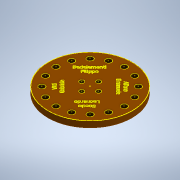
# Autodesk Inventor part: dischetto
Saved by Autodesk Inventor 2020.2 (Build 242310000, 310)
## iProperties
Created: 2020-02-12
Part Number: dischetto
Material: Legno(pioppo)
Document SubType Name: Modeling
Designer: socci
Density: 0.4 g/cm^3
Appearance: Default(1)
Mass: 18.3157 g
Surface Area: 156.78 cm^2
Volume: 45.7893 cm^3
Author: socci
Autodesk Inventor part; units mm, degrees
(part 1 of 3)
ref_plane "YZ Plane" through (0, 0, 0) normal (1, 0, 0) x (0, 1, 0)
ref_plane "XZ Plane" through (0, 0, 0) normal (0, 1, 0) x (-1, 0, 0)
ref_plane "XY Plane" through (0, 0, 0) normal (0, 0, 1) x (1, 0, 0)
sketch "Schizzo1" plane through (0, 0, 0) normal (0, 1, 0) x (-1, 0, 0)
  circle A0 centre (0, 0) radius 40
  dimension "d0" = 80
  constraints: 1 centre point, 1 coincident
  measures "d0" diameter of A0
extrude "Estrusione1" add sketch "Schizzo1" along normal blind 6
sketch "Schizzo2" plane through (0, 6, 0) normal (0, 1, 0) x (1, 0, 0)
  line L0 (0, -8) -> (0, 8)
  line L1 (0, -8) -> (16, -8) construction
  line L2 (-8, 0) -> (8, 0)
  line L3 (-8, 0) -> (8, 0) construction
  point P0 (0, 0)
  point P1 (0, 0)
  dimension "d4" = 16
  dimension "d5" = 90
  dimension "d6" = 16
  dimension "d7" = 0
  constraints: 8 end point, 3 horizontal, 2 equal length, 2 midpoint, 1 coincident, 1 vertical
  measures "d4" distance of L0.start L0.end
  measures "d5" angle of L1 L0
  measures "d6" distance of L2.start L2.end
  measures "d7" distance between parallel lines of L2 L3
hole "Foro1" at (-8, 6, 0) at (0, 6, 8) at (8, 6, 0) at (0, 6, -8) direction (0, -1, 0) diameter 4.2 end through all
sketch "Schizzo3" plane through (0, 6, 0) normal (0, 1, 0) x (1, 0, 0)
  line L0 (0, 0) -> (0, 32.5)
  point P0 (-12.4372, 30.0261)
  point P1 (-22.981, 22.981)
  point P2 (-30.0261, 12.4372)
  point P3 (-32.5, 0)
  point P4 (-30.0261, -12.4372)
  point P5 (-22.981, -22.981)
  point P6 (-12.4372, -30.0261)
  point P7 (0, -32.5)
  point P8 (12.4372, -30.0261)
  point P9 (22.981, -22.981)
  point P10 (30.0261, -12.4372)
  point P11 (32.5, 0)
  point P12 (30.0261, 12.4372)
  point P13 (22.981, 22.981)
  point P14 (12.4372, 30.0261)
  point P15 (24.3182, -23.5879)
  dimension "d15" = 32.5
  dimension "d19" = 360
  constraints: 2 end point, 1 coincident, 1 vertical, 17 other
  measures "d15" distance of L0.start L0.end
hole "Foro2" at (0, 6, -32.5) at (-30.0261, 6, 12.4372) at (-32.5, 6, 0) at (-30.0261, 6, -12.4372) at (-22.981, 6, -22.981) at (-12.4372, 6, -30.0261) at (12.4372, 6, -30.0261) at (22.981, 6, -22.981) at (30.0261, 6, -12.4372) at (32.5, 6, 0) at (30.0261, 6, 12.4372) at (22.981, 6, 22.981) at (12.4372, 6, 30.0261) at (0, 6, 32.5) at (-12.4372, 6, 30.0261) at (-22.981, 6, 22.981) direction (0, -1, 0) diameter 5.5 end through all clearance for "Vite a testa svasata piana ISO 2009/7046" size "M5" standard "ISO"
sketch "Schizzo4" plane through (0, 6, 0) normal (0, 1, 0) x (1, 0, 0)
  line L0 (-26.4914, 3.9695) -> (-4.5406, 25.9204) construction
  line L1 (-4.5406, 25.9204) -> (-2.2299, 23.6096) construction
  line L2 (-2.2299, 23.6096) -> (-24.1807, 1.6588) construction
  line L3 (-24.1807, 1.6588) -> (-26.4914, 3.9695) construction
  line L4 (9.0217, 26.78) -> (26.9135, 8.8882) construction
  line L5 (26.9135, 8.8882) -> (21.8287, 3.8034) construction
  line L6 (21.8287, 3.8034) -> (3.9369, 21.6952) construction
  line L7 (3.9369, 21.6952) -> (9.0217, 26.78) construction
  line L8 (-4.485, -26.3516) -> (-26.4359, -4.4008) construction
  line L9 (-26.4359, -4.4008) -> (-26.0745, -4.0394) construction
  line L10 (-26.0745, -4.0394) -> (-4.1237, -25.9903) construction
  line L11 (-4.1237, -25.9903) -> (-4.485, -26.3516) construction
  line L12 (23.0165, -8.2769) -> (5.176, -26.1174) construction
  line L13 (5.176, -26.1174) -> (2.8653, -23.8067) construction
  line L14 (2.8653, -23.8067) -> (20.7058, -5.9662) construction
  line L15 (20.7058, -5.9662) -> (23.0165, -8.2769) construction
  line L16 (0, 0) -> (32.9939, -32.9939) construction
  line L17 (0, 0) -> (46.6605, 0) construction
  line L18 (0, 0) -> (41.8573, 41.8573) construction
  line L19 (0, 0) -> (59.1951, 0) construction
  line L20 (0, 0) -> (-51.3067, 51.3067) construction
  line L21 (0, 0) -> (72.5586, 0) construction
  line L22 (0, 0) -> (-38.8019, -38.8019) construction
  line L23 (0, 0) -> (54.8741, 0) construction
  spline S0 degree 2 poles (-22.3396, 9.0274) (-22.1789, 8.8667) (-22.0549, 8.4981) (-22.0759, 8.3165) knots 0 0 0 1 2 2 2
  spline S1 degree 2 poles (-22.0759, 8.3165) (-22.1038, 8.0999) (-22.3012, 7.7419) (-22.5213, 7.5218) knots 0 0 0 1 2 2 2
  line L24 (-22.5213, 7.5218) -> (-23.1395, 6.9035)
  line L25 (-23.1395, 6.9035) -> (-25.2948, 9.0588)
  line L26 (-25.2948, 9.0588) -> (-24.7237, 9.6299)
  spline S2 degree 2 poles (-24.7237, 9.6299) (-24.4931, 9.8605) (-24.2329, 10.0613) (-24.0705, 10.1085) knots 0 0 0 1 2 2 2
  spline S3 degree 2 poles (-24.0705, 10.1085) (-23.8923, 10.1644) (-23.5849, 10.0701) (-23.4487, 9.9338) knots 0 0 0 1 2 2 2
  spline S4 degree 2 poles (-23.4487, 9.9338) (-23.2967, 9.7819) (-23.2164, 9.3802) (-23.2897, 9.1706) knots 0 0 0 1 2 2 2
  line L27 (-23.2897, 9.1706) -> (-23.2793, 9.1601)
  spline S5 degree 2 poles (-23.2793, 9.1601) (-23.0347, 9.2998) (-22.5457, 9.2335) (-22.3396, 9.0274) knots 0 0 0 1 2 2 2
  spline S6 degree 2 poles (-22.626, 8.7165) (-22.7483, 8.8387) (-22.9754, 8.9261) (-23.136, 8.8772) knots 0 0 0 1 2 2 2
  spline S7 degree 2 poles (-23.136, 8.8772) (-23.2391, 8.844) (-23.4207, 8.7042) (-23.5692, 8.5558) knots 0 0 0 1 2 2 2
  line L28 (-23.5692, 8.5558) -> (-23.8941, 8.2309)
  line L29 (-23.8941, 8.2309) -> (-23.0976, 7.4345)
  line L30 (-23.0976, 7.4345) -> (-22.8653, 7.6668)
  spline S8 degree 2 poles (-22.8653, 7.6668) (-22.6767, 7.8554) (-22.4951, 8.1069) (-22.4671, 8.2466) knots 0 0 0 1 2 2 2
  spline S9 degree 2 poles (-22.4671, 8.2466) (-22.4444, 8.3846) (-22.5125, 8.6029) (-22.626, 8.7165) knots 0 0 0 1 2 2 2
  spline S10 degree 2 poles (-23.7072, 9.595) (-23.784, 9.6718) (-23.9517, 9.7347) (-24.0425, 9.7103) knots 0 0 0 1 2 2 2
  spline S11 degree 2 poles (-24.0425, 9.7103) (-24.1508, 9.6788) (-24.3377, 9.5269) (-24.4896, 9.3749) knots 0 0 0 1 2 2 2
  line L31 (-24.4896, 9.3749) -> (-24.7638, 9.1007)
  line L32 (-24.7638, 9.1007) -> (-24.1333, 8.4702)
  line L33 (-24.1333, 8.4702) -> (-23.8085, 8.7951)
  spline S12 degree 2 poles (-23.8085, 8.7951) (-23.674, 8.9295) (-23.5744, 9.085) (-23.55, 9.1968) knots 0 0 0 1 2 2 2
  spline S13 degree 2 poles (-23.55, 9.1968) (-23.5255, 9.3051) (-23.6059, 9.4937) (-23.7072, 9.595) knots 0 0 0 1 2 2 2
  spline S14 degree 2 poles (-20.6839, 9.7015) (-20.6926, 9.6439) (-20.7171, 9.4448) (-20.7433, 9.3662) knots 0 0 0 1 2 2 2
  spline S15 degree 2 poles (-20.7433, 9.3662) (-20.7764, 9.2562) (-20.8708, 9.0815) (-20.993, 8.9592) knots 0 0 0 1 2 2 2
  spline S16 degree 2 poles (-20.993, 8.9592) (-21.0926, 8.8597) (-21.3476, 8.7549) (-21.4838, 8.7549) knots 0 0 0 1 2 2 2
  spline S17 degree 2 poles (-21.4838, 8.7549) (-21.6148, 8.7566) (-21.889, 8.8737) (-21.9973, 8.9819) knots 0 0 0 1 2 2 2
  spline S18 degree 2 poles (-21.9973, 8.9819) (-22.165, 9.1496) (-22.261, 9.5286) (-22.1754, 9.7504) knots 0 0 0 1 2 2 2
  spline S19 degree 2 poles (-22.1754, 9.7504) (-22.1021, 9.9495) (-21.779, 10.367) (-21.5764, 10.594) knots 0 0 0 1 2 2 2
  line L34 (-21.5764, 10.594) -> (-21.6288, 10.6464)
  spline S20 degree 2 poles (-21.6288, 10.6464) (-21.7231, 10.7407) (-21.8977, 10.8001) (-21.9833, 10.7809) knots 0 0 0 1 2 2 2
  spline S21 degree 2 poles (-21.9833, 10.7809) (-22.0689, 10.7617) (-22.2401, 10.6324) (-22.3204, 10.5521) knots 0 0 0 1 2 2 2
  spline S22 degree 2 poles (-22.3204, 10.5521) (-22.4147, 10.4578) (-22.6138, 10.1469) (-22.6872, 9.9653) knots 0 0 0 1 2 2 2
  line L35 (-22.6872, 9.9653) -> (-22.7029, 9.9495)
  line L36 (-22.7029, 9.9495) -> (-22.9806, 10.2272)
  spline S23 degree 2 poles (-22.9806, 10.2272) (-22.9265, 10.3233) (-22.6977, 10.6569) (-22.5597, 10.7949) knots 0 0 0 1 2 2 2
  spline S24 degree 2 poles (-22.5597, 10.7949) (-22.392, 10.9626) (-22.1108, 11.139) (-21.9519, 11.1617) knots 0 0 0 1 2 2 2
  spline S25 degree 2 poles (-21.9519, 11.1617) (-21.7964, 11.1844) (-21.4978, 11.0604) (-21.3458, 10.9084) knots 0 0 0 1 2 2 2
  line L37 (-21.3458, 10.9084) -> (-20.2402, 9.8028)
  line L38 (-20.2402, 9.8028) -> (-20.5127, 9.5304)
  line L39 (-20.5127, 9.5304) -> (-20.6839, 9.7015)
  line L40 (-20.9109, 9.9286) -> (-21.3598, 10.3775)
  spline S26 degree 2 poles (-21.3598, 10.3775) (-21.4489, 10.2709) (-21.7143, 9.946) (-21.779, 9.8255) knots 0 0 0 1 2 2 2
  spline S27 degree 2 poles (-21.779, 9.8255) (-21.8541, 9.6841) (-21.8576, 9.4046) (-21.7353, 9.2824) knots 0 0 0 1 2 2 2
  spline S28 degree 2 poles (-21.7353, 9.2824) (-21.5956, 9.1426) (-21.2969, 9.1583) (-21.1467, 9.3086) knots 0 0 0 1 2 2 2
  spline S29 degree 2 poles (-21.1467, 9.3086) (-21.0192, 9.4361) (-20.9197, 9.7557) (-20.9109, 9.9286) knots 0 0 0 1 2 2 2
  line L41 (-18.6142, 11.4289) -> (-18.8867, 11.1564)
  line L42 (-18.8867, 11.1564) -> (-19.0508, 11.3206)
  spline S30 degree 2 poles (-19.0508, 11.3206) (-19.0613, 11.2053) (-19.084, 11.0429) (-19.1172, 10.9503) knots 0 0 0 1 2 2 2
  spline S31 degree 2 poles (-19.1172, 10.9503) (-19.1469, 10.8647) (-19.2412, 10.711) (-19.3233, 10.629) knots 0 0 0 1 2 2 2
  spline S32 degree 2 poles (-19.3233, 10.629) (-19.456, 10.4962) (-19.7896, 10.3827) (-19.9748, 10.4106) knots 0 0 0 1 2 2 2
  spline S33 degree 2 poles (-19.9748, 10.4106) (-20.1599, 10.4386) (-20.5616, 10.6656) (-20.766, 10.87) knots 0 0 0 1 2 2 2
  spline S34 degree 2 poles (-20.766, 10.87) (-20.979, 11.0831) (-21.1799, 11.504) (-21.2009, 11.7171) knots 0 0 0 1 2 2 2
  spline S35 degree 2 poles (-21.2009, 11.7171) (-21.2166, 11.9109) (-21.0873, 12.2812) (-20.9493, 12.4192) knots 0 0 0 1 2 2 2
  spline S36 degree 2 poles (-20.9493, 12.4192) (-20.8288, 12.5397) (-20.5948, 12.6655) (-20.4394, 12.7091) knots 0 0 0 1 2 2 2
  line L43 (-20.4394, 12.7091) -> (-21.138, 13.4077)
  line L44 (-21.138, 13.4077) -> (-20.8655, 13.6802)
  line L45 (-20.8655, 13.6802) -> (-18.6142, 11.4289)
  line L46 (-19.2796, 11.5494) -> (-20.214, 12.4838)
  spline S37 degree 2 poles (-20.214, 12.4838) (-20.3642, 12.4314) (-20.5616, 12.3074) (-20.6542, 12.2148) knots 0 0 0 1 2 2 2
  spline S38 degree 2 poles (-20.6542, 12.2148) (-20.8638, 12.0052) (-20.7869, 11.4533) (-20.49, 11.1564) knots 0 0 0 1 2 2 2
  spline S39 degree 2 poles (-20.49, 11.1564) (-20.2036, 10.87) (-19.7198, 10.7495) (-19.5189, 10.9503) knots 0 0 0 1 2 2 2
  spline S40 degree 2 poles (-19.5189, 10.9503) (-19.4124, 11.0569) (-19.2936, 11.3712) (-19.2796, 11.5494) knots 0 0 0 1 2 2 2
  spline S41 degree 2 poles (-17.4894, 12.896) (-17.4981, 12.8384) (-17.5226, 12.6393) (-17.5488, 12.5607) knots 0 0 0 1 2 2 2
  spline S42 degree 2 poles (-17.5488, 12.5607) (-17.582, 12.4506) (-17.6763, 12.276) (-17.7985, 12.1537) knots 0 0 0 1 2 2 2
  spline S43 degree 2 poles (-17.7985, 12.1537) (-17.8981, 12.0542) (-18.1531, 11.9494) (-18.2893, 11.9494) knots 0 0 0 1 2 2 2
  spline S44 degree 2 poles (-18.2893, 11.9494) (-18.4203, 11.9511) (-18.6945, 12.0681) (-18.8028, 12.1764) knots 0 0 0 1 2 2 2
  spline S45 degree 2 poles (-18.8028, 12.1764) (-18.9705, 12.3441) (-19.0665, 12.7231) (-18.981, 12.9449) knots 0 0 0 1 2 2 2
  spline S46 degree 2 poles (-18.981, 12.9449) (-18.9076, 13.144) (-18.5845, 13.5614) (-18.3819, 13.7885) knots 0 0 0 1 2 2 2
  line L47 (-18.3819, 13.7885) -> (-18.4343, 13.8409)
  spline S47 degree 2 poles (-18.4343, 13.8409) (-18.5286, 13.9352) (-18.7033, 13.9946) (-18.7888, 13.9754) knots 0 0 0 1 2 2 2
  spline S48 degree 2 poles (-18.7888, 13.9754) (-18.8744, 13.9562) (-19.0456, 13.8269) (-19.1259, 13.7466) knots 0 0 0 1 2 2 2
  spline S49 degree 2 poles (-19.1259, 13.7466) (-19.2202, 13.6523) (-19.4194, 13.3414) (-19.4927, 13.1597) knots 0 0 0 1 2 2 2
  line L48 (-19.4927, 13.1597) -> (-19.5084, 13.144)
  line L49 (-19.5084, 13.144) -> (-19.7861, 13.4217)
  spline S50 degree 2 poles (-19.7861, 13.4217) (-19.732, 13.5178) (-19.5032, 13.8514) (-19.3652, 13.9893) knots 0 0 0 1 2 2 2
  spline S51 degree 2 poles (-19.3652, 13.9893) (-19.1975, 14.157) (-18.9163, 14.3334) (-18.7574, 14.3561) knots 0 0 0 1 2 2 2
  spline S52 degree 2 poles (-18.7574, 14.3561) (-18.602, 14.3788) (-18.3033, 14.2548) (-18.1513, 14.1029) knots 0 0 0 1 2 2 2
  line L50 (-18.1513, 14.1029) -> (-17.0458, 12.9973)
  line L51 (-17.0458, 12.9973) -> (-17.3182, 12.7248)
  line L52 (-17.3182, 12.7248) -> (-17.4894, 12.896)
  line L53 (-17.7165, 13.1231) -> (-18.1653, 13.5719)
  spline S53 degree 2 poles (-18.1653, 13.5719) (-18.2544, 13.4654) (-18.5199, 13.1405) (-18.5845, 13.02) knots 0 0 0 1 2 2 2
  spline S54 degree 2 poles (-18.5845, 13.02) (-18.6596, 12.8785) (-18.6631, 12.5991) (-18.5408, 12.4768) knots 0 0 0 1 2 2 2
  spline S55 degree 2 poles (-18.5408, 12.4768) (-18.4011, 12.3371) (-18.1024, 12.3528) (-17.9522, 12.503) knots 0 0 0 1 2 2 2
  spline S56 degree 2 poles (-17.9522, 12.503) (-17.8247, 12.6305) (-17.7252, 12.9501) (-17.7165, 13.1231) knots 0 0 0 1 2 2 2
  line L54 (-16.3856, 13.6575) -> (-16.658, 13.385)
  line L55 (-16.658, 13.385) -> (-18.9094, 15.6364)
  line L56 (-18.9094, 15.6364) -> (-18.6369, 15.9088)
  line L57 (-18.6369, 15.9088) -> (-16.3856, 13.6575)
  spline S57 degree 2 poles (-15.2555, 15.1299) (-15.2643, 15.0722) (-15.2887, 14.8731) (-15.3149, 14.7945) knots 0 0 0 1 2 2 2
  spline S58 degree 2 poles (-15.3149, 14.7945) (-15.3481, 14.6845) (-15.4424, 14.5098) (-15.5647, 14.3876) knots 0 0 0 1 2 2 2
  spline S59 degree 2 poles (-15.5647, 14.3876) (-15.6642, 14.288) (-15.9192, 14.1832) (-16.0555, 14.1832) knots 0 0 0 1 2 2 2
  spline S60 degree 2 poles (-16.0555, 14.1832) (-16.1865, 14.185) (-16.4607, 14.302) (-16.569, 14.4103) knots 0 0 0 1 2 2 2
  spline S61 degree 2 poles (-16.569, 14.4103) (-16.7366, 14.5779) (-16.8327, 14.9569) (-16.7471, 15.1788) knots 0 0 0 1 2 2 2
  spline S62 degree 2 poles (-16.7471, 15.1788) (-16.6738, 15.3779) (-16.3506, 15.7953) (-16.148, 16.0223) knots 0 0 0 1 2 2 2
  line L58 (-16.148, 16.0223) -> (-16.2004, 16.0747)
  spline S63 degree 2 poles (-16.2004, 16.0747) (-16.2948, 16.1691) (-16.4694, 16.2284) (-16.555, 16.2092) knots 0 0 0 1 2 2 2
  spline S64 degree 2 poles (-16.555, 16.2092) (-16.6406, 16.19) (-16.8117, 16.0608) (-16.8921, 15.9804) knots 0 0 0 1 2 2 2
  spline S65 degree 2 poles (-16.8921, 15.9804) (-16.9864, 15.8861) (-17.1855, 15.5752) (-17.2589, 15.3936) knots 0 0 0 1 2 2 2
  line L59 (-17.2589, 15.3936) -> (-17.2746, 15.3779)
  line L60 (-17.2746, 15.3779) -> (-17.5523, 15.6556)
  spline S66 degree 2 poles (-17.5523, 15.6556) (-17.4981, 15.7516) (-17.2693, 16.0852) (-17.1314, 16.2232) knots 0 0 0 1 2 2 2
  spline S67 degree 2 poles (-17.1314, 16.2232) (-16.9637, 16.3909) (-16.6825, 16.5673) (-16.5236, 16.59) knots 0 0 0 1 2 2 2
  spline S68 degree 2 poles (-16.5236, 16.59) (-16.3681, 16.6127) (-16.0694, 16.4887) (-15.9175, 16.3367) knots 0 0 0 1 2 2 2
  line L61 (-15.9175, 16.3367) -> (-14.8119, 15.2312)
  line L62 (-14.8119, 15.2312) -> (-15.0844, 14.9587)
  line L63 (-15.0844, 14.9587) -> (-15.2555, 15.1299)
  line L64 (-15.4826, 15.3569) -> (-15.9315, 15.8058)
  spline S69 degree 2 poles (-15.9315, 15.8058) (-16.0205, 15.6992) (-16.286, 15.3744) (-16.3506, 15.2539) knots 0 0 0 1 2 2 2
  spline S70 degree 2 poles (-16.3506, 15.2539) (-16.4257, 15.1124) (-16.4292, 14.8329) (-16.307, 14.7107) knots 0 0 0 1 2 2 2
  spline S71 degree 2 poles (-16.307, 14.7107) (-16.1673, 14.571) (-15.8686, 14.5867) (-15.7184, 14.7369) knots 0 0 0 1 2 2 2
  spline S72 degree 2 poles (-15.7184, 14.7369) (-15.5909, 14.8644) (-15.4913, 15.184) (-15.4826, 15.3569) knots 0 0 0 1 2 2 2
  line L65 (-12.5955, 17.4475) -> (-13.5317, 18.3837)
  spline S73 degree 2 poles (-13.5317, 18.3837) (-13.6435, 18.4955) (-13.8513, 18.6684) (-13.9316, 18.6928) knots 0 0 0 1 2 2 2
  spline S74 degree 2 poles (-13.9316, 18.6928) (-14.0172, 18.7225) (-14.1797, 18.6719) (-14.2722, 18.5793) knots 0 0 0 1 2 2 2
  spline S75 degree 2 poles (-14.2722, 18.5793) (-14.3561, 18.4955) (-14.4451, 18.2003) (-14.4486, 18.0012) knots 0 0 0 1 2 2 2
  spline S76 degree 2 poles (-14.4486, 18.0012) (-14.4224, 17.9785) (-14.3508, 17.9139) (-14.3054, 17.8685) knots 0 0 0 1 2 2 2
  line L66 (-14.3054, 17.8685) -> (-13.24, 16.8031)
  line L67 (-13.24, 16.8031) -> (-13.5125, 16.5306)
  line L68 (-13.5125, 16.5306) -> (-14.4486, 17.4668)
  spline S77 degree 2 poles (-14.4486, 17.4668) (-14.5604, 17.5785) (-14.7683, 17.7514) (-14.8486, 17.7759) knots 0 0 0 1 2 2 2
  spline S78 degree 2 poles (-14.8486, 17.7759) (-14.9342, 17.8056) (-15.0966, 17.7549) (-15.1892, 17.6624) knots 0 0 0 1 2 2 2
  spline S79 degree 2 poles (-15.1892, 17.6624) (-15.2765, 17.575) (-15.3603, 17.2711) (-15.3656, 17.0947) knots 0 0 0 1 2 2 2
  line L69 (-15.3656, 17.0947) -> (-14.157, 15.8861)
  line L70 (-14.157, 15.8861) -> (-14.4294, 15.6137)
  line L71 (-14.4294, 15.6137) -> (-16.0467, 17.231)
  line L72 (-16.0467, 17.231) -> (-15.7743, 17.5034)
  line L73 (-15.7743, 17.5034) -> (-15.5961, 17.3253)
  spline S80 degree 2 poles (-15.5961, 17.3253) (-15.5961, 17.5384) (-15.5036, 17.865) (-15.3778, 17.9907) knots 0 0 0 1 2 2 2
  spline S81 degree 2 poles (-15.3778, 17.9907) (-15.2346, 18.1339) (-14.8818, 18.2248) (-14.6757, 18.1339) knots 0 0 0 1 2 2 2
  spline S82 degree 2 poles (-14.6757, 18.1339) (-14.6897, 18.3959) (-14.5971, 18.7714) (-14.4609, 18.9077) knots 0 0 0 1 2 2 2
  spline S83 degree 2 poles (-14.4609, 18.9077) (-14.3561, 19.0125) (-14.1203, 19.119) (-13.984, 19.1085) knots 0 0 0 1 2 2 2
  spline S84 degree 2 poles (-13.984, 19.1085) (-13.8461, 19.0998) (-13.5544, 18.9513) (-13.3885, 18.7854) knots 0 0 0 1 2 2 2
  line L74 (-13.3885, 18.7854) -> (-12.3231, 17.72)
  line L75 (-12.3231, 17.72) -> (-12.5955, 17.4475)
  spline S85 degree 2 poles (-11.2018, 18.768) (-11.5895, 18.3802) (-12.4506, 18.3889) (-12.8523, 18.7907) knots 0 0 0 1 2 2 2
  spline S86 degree 2 poles (-12.8523, 18.7907) (-13.247, 19.1854) (-13.3011, 20.0674) (-12.9675, 20.401) knots 0 0 0 1 2 2 2
  spline S87 degree 2 poles (-12.9675, 20.401) (-12.8173, 20.5512) (-12.4977, 20.6962) (-12.3196, 20.6892) knots 0 0 0 1 2 2 2
  spline S88 degree 2 poles (-12.3196, 20.6892) (-12.1397, 20.6839) (-11.7799, 20.5093) (-11.586, 20.3154) knots 0 0 0 1 2 2 2
  line L76 (-11.586, 20.3154) -> (-11.4376, 20.1669)
  line L77 (-11.4376, 20.1669) -> (-12.5571, 19.0474)
  spline S89 degree 2 poles (-12.5571, 19.0474) (-12.2759, 18.7662) (-11.6943, 18.7505) (-11.4428, 19.002) knots 0 0 0 1 2 2 2
  spline S90 degree 2 poles (-11.4428, 19.002) (-11.3537, 19.0911) (-11.221, 19.3041) (-11.1826, 19.4054) knots 0 0 0 1 2 2 2
  spline S91 degree 2 poles (-11.1826, 19.4054) (-11.1441, 19.5137) (-11.104, 19.6762) (-11.0987, 19.7373) knots 0 0 0 1 2 2 2
  line L78 (-11.0987, 19.7373) -> (-11.083, 19.753)
  line L79 (-11.083, 19.753) -> (-10.7861, 19.4561)
  spline S92 degree 2 poles (-10.7861, 19.4561) (-10.814, 19.3897) (-10.9014, 19.1906) (-10.9415, 19.119) knots 0 0 0 1 2 2 2
  spline S93 degree 2 poles (-10.9415, 19.119) (-10.9974, 19.0177) (-11.104, 18.8658) (-11.2018, 18.768) knots 0 0 0 1 2 2 2
  spline S94 degree 2 poles (-11.9109, 20.1093) (-12.0244, 20.2159) (-12.2305, 20.3311) (-12.3283, 20.3416) knots 0 0 0 1 2 2 2
  spline S95 degree 2 poles (-12.3283, 20.3416) (-12.4366, 20.3556) (-12.6497, 20.2717) (-12.7597, 20.1617) knots 0 0 0 1 2 2 2
  spline S96 degree 2 poles (-12.7597, 20.1617) (-12.868, 20.0534) (-12.9553, 19.8368) (-12.9553, 19.7111) knots 0 0 0 1 2 2 2
  spline S97 degree 2 poles (-12.9553, 19.7111) (-12.9518, 19.5853) (-12.8593, 19.367) (-12.7649, 19.2552) knots 0 0 0 1 2 2 2
  line L80 (-12.7649, 19.2552) -> (-11.9109, 20.1093)
  line L81 (-9.1111, 20.9319) -> (-9.3836, 20.6595)
  line L82 (-9.3836, 20.6595) -> (-10.3058, 21.5817)
  spline S98 degree 2 poles (-10.3058, 21.5817) (-10.4176, 21.6934) (-10.6306, 21.8646) (-10.7197, 21.8908) knots 0 0 0 1 2 2 2
  spline S99 degree 2 poles (-10.7197, 21.8908) (-10.814, 21.9188) (-10.9922, 21.8594) (-11.0935, 21.7581) knots 0 0 0 1 2 2 2
  spline S100 degree 2 poles (-11.0935, 21.7581) (-11.1948, 21.6568) (-11.3013, 21.3337) (-11.317, 21.1433) knots 0 0 0 1 2 2 2
  line L83 (-11.317, 21.1433) -> (-10.1084, 19.9347)
  line L84 (-10.1084, 19.9347) -> (-10.3809, 19.6622)
  line L85 (-10.3809, 19.6622) -> (-11.9982, 21.2795)
  line L86 (-11.9982, 21.2795) -> (-11.7257, 21.552)
  line L87 (-11.7257, 21.552) -> (-11.5458, 21.3721)
  spline S101 degree 2 poles (-11.5458, 21.3721) (-11.5336, 21.6044) (-11.4131, 21.9554) (-11.2804, 22.0882) knots 0 0 0 1 2 2 2
  spline S102 degree 2 poles (-11.2804, 22.0882) (-11.0428, 22.3257) (-10.4595, 22.2803) (-10.1608, 21.9816) knots 0 0 0 1 2 2 2
  line L88 (-10.1608, 21.9816) -> (-9.1111, 20.9319)
  spline S103 degree 2 poles (-8.2082, 21.772) (-8.43, 21.5502) (-8.933, 21.5537) (-9.2072, 21.8279) knots 0 0 0 1 2 2 2
  line L89 (-9.2072, 21.8279) -> (-10.1032, 22.7239)
  line L90 (-10.1032, 22.7239) -> (-10.2866, 22.5405)
  line L91 (-10.2866, 22.5405) -> (-10.5119, 22.7658)
  line L92 (-10.5119, 22.7658) -> (-10.3285, 22.9492)
  line L93 (-10.3285, 22.9492) -> (-10.7931, 23.4138)
  line L94 (-10.7931, 23.4138) -> (-10.5206, 23.6863)
  line L95 (-10.5206, 23.6863) -> (-10.056, 23.2217)
  line L96 (-10.056, 23.2217) -> (-9.5548, 23.723)
  line L97 (-9.5548, 23.723) -> (-9.3294, 23.4976)
  line L98 (-9.3294, 23.4976) -> (-9.8307, 22.9964)
  line L99 (-9.8307, 22.9964) -> (-9.0605, 22.2261)
  spline S104 degree 2 poles (-9.0605, 22.2261) (-8.9382, 22.1039) (-8.795, 21.9781) (-8.7077, 21.9502) knots 0 0 0 1 2 2 2
  spline S105 degree 2 poles (-8.7077, 21.9502) (-8.6326, 21.924) (-8.4719, 21.9834) (-8.3776, 22.0777) knots 0 0 0 1 2 2 2
  spline S106 degree 2 poles (-8.3776, 22.0777) (-8.3112, 22.1441) (-8.2274, 22.3082) (-8.2116, 22.3484) knots 0 0 0 1 2 2 2
  line L100 (-8.2116, 22.3484) -> (-8.1959, 22.3641)
  line L101 (-8.1959, 22.3641) -> (-7.9514, 22.1196)
  spline S107 degree 2 poles (-7.9514, 22.1196) (-8.0073, 22.0218) (-8.14, 21.8402) (-8.2082, 21.772) knots 0 0 0 1 2 2 2
  line L102 (-7.4589, 22.5842) -> (-7.7313, 22.3117)
  line L103 (-7.7313, 22.3117) -> (-9.3487, 23.9291)
  line L104 (-9.3487, 23.9291) -> (-9.0762, 24.2015)
  line L105 (-9.0762, 24.2015) -> (-7.4589, 22.5842)
  line L106 (-9.326, 24.4897) -> (-9.6351, 24.1806)
  line L107 (-9.6351, 24.1806) -> (-9.918, 24.4635)
  line L108 (-9.918, 24.4635) -> (-9.6089, 24.7726)
  line L109 (-9.6089, 24.7726) -> (-9.326, 24.4897)
  line L110 (-16.3834, 10.363) -> (-17.3859, 9.3605)
  line L111 (-17.3859, 9.3605) -> (-16.7781, 8.7527)
  line L112 (-16.7781, 8.7527) -> (-15.8175, 9.7133)
  line L113 (-15.8175, 9.7133) -> (-15.5625, 9.4583)
  line L114 (-15.5625, 9.4583) -> (-16.5231, 8.4977)
  line L115 (-16.5231, 8.4977) -> (-15.4857, 7.4603)
  line L116 (-15.4857, 7.4603) -> (-15.7721, 7.1738)
  line L117 (-15.7721, 7.1738) -> (-17.9274, 9.3291)
  line L118 (-17.9274, 9.3291) -> (-16.6384, 10.618)
  line L119 (-16.6384, 10.618) -> (-16.3834, 10.363)
  line L120 (-13.9696, 8.9763) -> (-14.2421, 8.7038)
  line L121 (-14.2421, 8.7038) -> (-15.8594, 10.3211)
  line L122 (-15.8594, 10.3211) -> (-15.587, 10.5936)
  line L123 (-15.587, 10.5936) -> (-13.9696, 8.9763)
  line L124 (-15.8367, 10.8818) -> (-16.1459, 10.5726)
  line L125 (-16.1459, 10.5726) -> (-16.4288, 10.8556)
  line L126 (-16.4288, 10.8556) -> (-16.1197, 11.1647)
  line L127 (-16.1197, 11.1647) -> (-15.8367, 10.8818)
  line L128 (-13.292, 9.6539) -> (-13.5644, 9.3815)
  line L129 (-13.5644, 9.3815) -> (-15.8158, 11.6328)
  line L130 (-15.8158, 11.6328) -> (-15.5433, 11.9053)
  line L131 (-15.5433, 11.9053) -> (-13.292, 9.6539)
  line L132 (-12.6143, 10.3316) -> (-12.8868, 10.0591)
  line L133 (-12.8868, 10.0591) -> (-14.5041, 11.6765)
  line L134 (-14.5041, 11.6765) -> (-14.2316, 11.9489)
  line L135 (-14.2316, 11.9489) -> (-12.6143, 10.3316)
  line L136 (-14.4814, 12.2371) -> (-14.7905, 11.928)
  line L137 (-14.7905, 11.928) -> (-15.0735, 12.2109)
  line L138 (-15.0735, 12.2109) -> (-14.7643, 12.5201)
  line L139 (-14.7643, 12.5201) -> (-14.4814, 12.2371)
  spline S108 degree 2 poles (-11.7113, 12.9392) (-11.3061, 12.534) (-11.2136, 11.6695) (-11.5087, 11.3743) knots 0 0 0 1 2 2 2
  spline S109 degree 2 poles (-11.5087, 11.3743) (-11.6292, 11.2538) (-11.8703, 11.1245) (-12.024, 11.0861) knots 0 0 0 1 2 2 2
  line L140 (-12.024, 11.0861) -> (-11.3463, 10.4085)
  line L141 (-11.3463, 10.4085) -> (-11.6188, 10.136)
  line L142 (-11.6188, 10.136) -> (-13.8317, 12.3489)
  line L143 (-13.8317, 12.3489) -> (-13.5592, 12.6214)
  line L144 (-13.5592, 12.6214) -> (-13.3898, 12.4519)
  spline S110 degree 2 poles (-13.3898, 12.4519) (-13.381, 12.6458) (-13.2553, 13.0161) (-13.1103, 13.161) knots 0 0 0 1 2 2 2
  spline S111 degree 2 poles (-13.1103, 13.161) (-12.8326, 13.4387) (-12.0816, 13.3095) (-11.7113, 12.9392) knots 0 0 0 1 2 2 2
  spline S112 degree 2 poles (-11.9611, 12.6266) (-12.2388, 12.9043) (-12.7208, 13.0335) (-12.9182, 12.8362) knots 0 0 0 1 2 2 2
  spline S113 degree 2 poles (-12.9182, 12.8362) (-13.0335, 12.7209) (-13.147, 12.4013) (-13.1627, 12.2249) knots 0 0 0 1 2 2 2
  line L145 (-13.1627, 12.2249) -> (-12.244, 11.3062)
  spline S114 degree 2 poles (-12.244, 11.3062) (-12.0868, 11.3621) (-11.8965, 11.4756) (-11.7987, 11.5734) knots 0 0 0 1 2 2 2
  spline S115 degree 2 poles (-11.7987, 11.5734) (-11.5873, 11.7847) (-11.6642, 12.3297) (-11.9611, 12.6266) knots 0 0 0 1 2 2 2
  spline S116 degree 2 poles (-10.0731, 14.5775) (-9.6678, 14.1723) (-9.5753, 13.3078) (-9.8704, 13.0126) knots 0 0 0 1 2 2 2
  spline S117 degree 2 poles (-9.8704, 13.0126) (-9.991, 12.8921) (-10.232, 12.7628) (-10.3857, 12.7244) knots 0 0 0 1 2 2 2
  line L146 (-10.3857, 12.7244) -> (-9.708, 12.0467)
  line L147 (-9.708, 12.0467) -> (-9.9805, 11.7743)
  line L148 (-9.9805, 11.7743) -> (-12.1934, 13.9872)
  line L149 (-12.1934, 13.9872) -> (-11.9209, 14.2596)
  line L150 (-11.9209, 14.2596) -> (-11.7515, 14.0902)
  spline S118 degree 2 poles (-11.7515, 14.0902) (-11.7428, 14.2841) (-11.617, 14.6544) (-11.4721, 14.7993) knots 0 0 0 1 2 2 2
  spline S119 degree 2 poles (-11.4721, 14.7993) (-11.1943, 15.077) (-10.4433, 14.9478) (-10.0731, 14.5775) knots 0 0 0 1 2 2 2
  spline S120 degree 2 poles (-10.3228, 14.2649) (-10.6005, 14.5426) (-11.0826, 14.6718) (-11.2799, 14.4745) knots 0 0 0 1 2 2 2
  spline S121 degree 2 poles (-11.2799, 14.4745) (-11.3952, 14.3592) (-11.5087, 14.0396) (-11.5244, 13.8632) knots 0 0 0 1 2 2 2
  line L151 (-11.5244, 13.8632) -> (-10.6058, 12.9445)
  spline S122 degree 2 poles (-10.6058, 12.9445) (-10.4486, 13.0004) (-10.2582, 13.1139) (-10.1604, 13.2117) knots 0 0 0 1 2 2 2
  spline S123 degree 2 poles (-10.1604, 13.2117) (-9.949, 13.423) (-10.0259, 13.968) (-10.3228, 14.2649) knots 0 0 0 1 2 2 2
  spline S124 degree 2 poles (-8.4173, 16.1459) (-8.0086, 15.7372) (-7.9562, 14.8989) (-8.2846, 14.5705) knots 0 0 0 1 2 2 2
  spline S125 degree 2 poles (-8.2846, 14.5705) (-8.6217, 14.2334) (-9.467, 14.3068) (-9.8617, 14.7015) knots 0 0 0 1 2 2 2
  spline S126 degree 2 poles (-9.8617, 14.7015) (-10.2669, 15.1067) (-10.3176, 15.9538) (-9.9927, 16.2787) knots 0 0 0 1 2 2 2
  spline S127 degree 2 poles (-9.9927, 16.2787) (-9.6644, 16.607) (-8.8243, 16.5529) (-8.4173, 16.1459) knots 0 0 0 1 2 2 2
  spline S128 degree 2 poles (-8.6985, 15.8647) (-9.0129, 16.1791) (-9.5473, 16.256) (-9.7587, 16.0446) knots 0 0 0 1 2 2 2
  spline S129 degree 2 poles (-9.7587, 16.0446) (-9.97, 15.8333) (-9.8949, 15.2971) (-9.5805, 14.9827) knots 0 0 0 1 2 2 2
  spline S130 degree 2 poles (-9.5805, 14.9827) (-9.2749, 14.6771) (-8.7299, 14.5932) (-8.5186, 14.8046) knots 0 0 0 1 2 2 2
  spline S131 degree 2 poles (-8.5186, 14.8046) (-8.309, 15.0141) (-8.3876, 15.5538) (-8.6985, 15.8647) knots 0 0 0 1 2 2 2
  line L152 (11.9676, 20.078) -> (14.8495, 21.5066)
  line L153 (14.8495, 21.5066) -> (15.2023, 21.1538)
  line L154 (15.2023, 21.1538) -> (13.7736, 18.272)
  line L155 (13.7736, 18.272) -> (13.4714, 18.5742)
  line L156 (13.4714, 18.5742) -> (13.8784, 19.3723)
  line L157 (13.8784, 19.3723) -> (13.0558, 20.195)
  line L158 (13.0558, 20.195) -> (12.2576, 19.788)
  line L159 (12.2576, 19.788) -> (11.9676, 20.078)
  line L160 (14.0443, 19.6955) -> (14.7255, 21.0438)
  line L161 (14.7255, 21.0438) -> (13.3789, 20.3609)
  line L162 (13.3789, 20.3609) -> (14.0443, 19.6955)
  line L163 (14.2347, 17.8109) -> (13.9622, 18.0834)
  line L164 (13.9622, 18.0834) -> (16.2135, 20.3347)
  line L165 (16.2135, 20.3347) -> (16.486, 20.0622)
  line L166 (16.486, 20.0622) -> (14.2347, 17.8109)
  line L167 (17.4746, 18.5497) -> (17.4606, 18.5637)
  spline S132 degree 2 poles (17.4606, 18.5637) (17.4379, 18.6143) (17.3261, 18.775) (17.272, 18.8292) knots 0 0 0 1 2 2 2
  spline S133 degree 2 poles (17.272, 18.8292) (17.1008, 19.0003) (16.8004, 18.9933) (16.5978, 18.7907) knots 0 0 0 1 2 2 2
  line L168 (16.5978, 18.7907) -> (16.5436, 18.7366)
  line L169 (16.5436, 18.7366) -> (16.9943, 18.286)
  line L170 (16.9943, 18.286) -> (16.7689, 18.0607)
  line L171 (16.7689, 18.0607) -> (16.3271, 18.5025)
  line L172 (16.3271, 18.5025) -> (14.9351, 17.1105)
  line L173 (14.9351, 17.1105) -> (14.6626, 17.383)
  line L174 (14.6626, 17.383) -> (16.0546, 18.775)
  line L175 (16.0546, 18.775) -> (15.8712, 18.9584)
  line L176 (15.8712, 18.9584) -> (16.0965, 19.1837)
  line L177 (16.0965, 19.1837) -> (16.2799, 19.0003)
  line L178 (16.2799, 19.0003) -> (16.3341, 19.0545)
  spline S134 degree 2 poles (16.3341, 19.0545) (16.624, 19.3444) (17.2091, 19.3671) (17.4711, 19.1051) knots 0 0 0 1 2 2 2
  spline S135 degree 2 poles (17.4711, 19.1051) (17.5462, 19.03) (17.6754, 18.8693) (17.7243, 18.7995) knots 0 0 0 1 2 2 2
  line L179 (17.7243, 18.7995) -> (17.4746, 18.5497)
  spline S136 degree 2 poles (16.6502, 15.7377) (16.5925, 15.7465) (16.3934, 15.7709) (16.3148, 15.7971) knots 0 0 0 1 2 2 2
  spline S137 degree 2 poles (16.3148, 15.7971) (16.2048, 15.8303) (16.0302, 15.9246) (15.9079, 16.0469) knots 0 0 0 1 2 2 2
  spline S138 degree 2 poles (15.9079, 16.0469) (15.8083, 16.1464) (15.7035, 16.4014) (15.7035, 16.5377) knots 0 0 0 1 2 2 2
  spline S139 degree 2 poles (15.7035, 16.5377) (15.7053, 16.6687) (15.8223, 16.9429) (15.9306, 17.0512) knots 0 0 0 1 2 2 2
  spline S140 degree 2 poles (15.9306, 17.0512) (16.0983, 17.2188) (16.4773, 17.3149) (16.6991, 17.2293) knots 0 0 0 1 2 2 2
  spline S141 degree 2 poles (16.6991, 17.2293) (16.8982, 17.1559) (17.3156, 16.8328) (17.5427, 16.6302) knots 0 0 0 1 2 2 2
  line L180 (17.5427, 16.6302) -> (17.5951, 16.6826)
  spline S142 degree 2 poles (17.5951, 16.6826) (17.6894, 16.7769) (17.7488, 16.9516) (17.7296, 17.0372) knots 0 0 0 1 2 2 2
  spline S143 degree 2 poles (17.7296, 17.0372) (17.7103, 17.1228) (17.5811, 17.2939) (17.5008, 17.3743) knots 0 0 0 1 2 2 2
  spline S144 degree 2 poles (17.5008, 17.3743) (17.4064, 17.4686) (17.0956, 17.6677) (16.9139, 17.741) knots 0 0 0 1 2 2 2
  line L181 (16.9139, 17.741) -> (16.8982, 17.7568)
  line L182 (16.8982, 17.7568) -> (17.1759, 18.0345)
  spline S145 degree 2 poles (17.1759, 18.0345) (17.272, 17.9803) (17.6056, 17.7515) (17.7435, 17.6135) knots 0 0 0 1 2 2 2
  spline S146 degree 2 poles (17.7435, 17.6135) (17.9112, 17.4459) (18.0876, 17.1647) (18.1103, 17.0057) knots 0 0 0 1 2 2 2
  spline S147 degree 2 poles (18.1103, 17.0057) (18.133, 16.8503) (18.009, 16.5516) (17.8571, 16.3997) knots 0 0 0 1 2 2 2
  line L183 (17.8571, 16.3997) -> (16.7515, 15.2941)
  line L184 (16.7515, 15.2941) -> (16.479, 15.5666)
  line L185 (16.479, 15.5666) -> (16.6502, 15.7377)
  line L186 (16.8772, 15.9648) -> (17.3261, 16.4137)
  spline S148 degree 2 poles (17.3261, 16.4137) (17.2196, 16.5027) (16.8947, 16.7682) (16.7742, 16.8328) knots 0 0 0 1 2 2 2
  spline S149 degree 2 poles (16.7742, 16.8328) (16.6327, 16.9079) (16.3533, 16.9114) (16.231, 16.7892) knots 0 0 0 1 2 2 2
  spline S150 degree 2 poles (16.231, 16.7892) (16.0913, 16.6494) (16.107, 16.3508) (16.2572, 16.2006) knots 0 0 0 1 2 2 2
  spline S151 degree 2 poles (16.2572, 16.2006) (16.3847, 16.0731) (16.7043, 15.9735) (16.8772, 15.9648) knots 0 0 0 1 2 2 2
  line L187 (18.4037, 13.6419) -> (18.1313, 13.9143)
  line L188 (18.1313, 13.9143) -> (19.0535, 14.8365)
  spline S152 degree 2 poles (19.0535, 14.8365) (19.1652, 14.9483) (19.3364, 15.1614) (19.3626, 15.2504) knots 0 0 0 1 2 2 2
  spline S153 degree 2 poles (19.3626, 15.2504) (19.3905, 15.3448) (19.3312, 15.5229) (19.2299, 15.6242) knots 0 0 0 1 2 2 2
  spline S154 degree 2 poles (19.2299, 15.6242) (19.1286, 15.7255) (18.8054, 15.8321) (18.6151, 15.8478) knots 0 0 0 1 2 2 2
  line L189 (18.6151, 15.8478) -> (17.4064, 14.6391)
  line L190 (17.4064, 14.6391) -> (17.134, 14.9116)
  line L191 (17.134, 14.9116) -> (18.7513, 16.5289)
  line L192 (18.7513, 16.5289) -> (19.0238, 16.2565)
  line L193 (19.0238, 16.2565) -> (18.8439, 16.0766)
  spline S155 degree 2 poles (18.8439, 16.0766) (19.0762, 16.0643) (19.4272, 15.9438) (19.56, 15.8111) knots 0 0 0 1 2 2 2
  spline S156 degree 2 poles (19.56, 15.8111) (19.7975, 15.5736) (19.7521, 14.9902) (19.4534, 14.6915) knots 0 0 0 1 2 2 2
  line L194 (19.4534, 14.6915) -> (18.4037, 13.6419)
  spline S157 degree 2 poles (20.924, 12.7389) (20.5153, 12.3302) (19.677, 12.2778) (19.3486, 12.6061) knots 0 0 0 1 2 2 2
  spline S158 degree 2 poles (19.3486, 12.6061) (19.0115, 12.9432) (19.0849, 13.7886) (19.4796, 14.1833) knots 0 0 0 1 2 2 2
  spline S159 degree 2 poles (19.4796, 14.1833) (19.8848, 14.5885) (20.7319, 14.6391) (21.0568, 14.3143) knots 0 0 0 1 2 2 2
  spline S160 degree 2 poles (21.0568, 14.3143) (21.3851, 13.9859) (21.331, 13.1458) (20.924, 12.7389) knots 0 0 0 1 2 2 2
  spline S161 degree 2 poles (20.6428, 13.0201) (20.9572, 13.3345) (21.0341, 13.8689) (20.8227, 14.0802) knots 0 0 0 1 2 2 2
  spline S162 degree 2 poles (20.8227, 14.0802) (20.6114, 14.2916) (20.0752, 14.2165) (19.7608, 13.9021) knots 0 0 0 1 2 2 2
  spline S163 degree 2 poles (19.7608, 13.9021) (19.4552, 13.5964) (19.3713, 13.0515) (19.5827, 12.8402) knots 0 0 0 1 2 2 2
  spline S164 degree 2 poles (19.5827, 12.8402) (19.7923, 12.6306) (20.3319, 12.7092) (20.6428, 13.0201) knots 0 0 0 1 2 2 2
  line L195 (6.3546, 18.5938) -> (8.5099, 20.7491)
  line L196 (8.5099, 20.7491) -> (9.8582, 19.4007)
  line L197 (9.8582, 19.4007) -> (9.6032, 19.1457)
  line L198 (9.6032, 19.1457) -> (8.5413, 20.2076)
  line L199 (8.5413, 20.2076) -> (7.951, 19.6173)
  line L200 (7.951, 19.6173) -> (8.9413, 18.627)
  line L201 (8.9413, 18.627) -> (8.6863, 18.372)
  line L202 (8.6863, 18.372) -> (7.696, 19.3623)
  line L203 (7.696, 19.3623) -> (6.8961, 18.5624)
  line L204 (6.8961, 18.5624) -> (7.958, 17.5005)
  line L205 (7.958, 17.5005) -> (7.703, 17.2455)
  line L206 (7.703, 17.2455) -> (6.3546, 18.5938)
  line L207 (9.8303, 15.1181) -> (10.7664, 16.0543)
  spline S165 degree 2 poles (10.7664, 16.0543) (10.8782, 16.1661) (11.0511, 16.3739) (11.0756, 16.4543) knots 0 0 0 1 2 2 2
  spline S166 degree 2 poles (11.0756, 16.4543) (11.1053, 16.5398) (11.0546, 16.7023) (10.9621, 16.7948) knots 0 0 0 1 2 2 2
  spline S167 degree 2 poles (10.9621, 16.7948) (10.8782, 16.8787) (10.5831, 16.9678) (10.3839, 16.9712) knots 0 0 0 1 2 2 2
  spline S168 degree 2 poles (10.3839, 16.9712) (10.3612, 16.9451) (10.2966, 16.8734) (10.2512, 16.828) knots 0 0 0 1 2 2 2
  line L208 (10.2512, 16.828) -> (9.1858, 15.7626)
  line L209 (9.1858, 15.7626) -> (8.9133, 16.0351)
  line L210 (8.9133, 16.0351) -> (9.8495, 16.9712)
  spline S169 degree 2 poles (9.8495, 16.9712) (9.9613, 17.083) (10.1342, 17.2909) (10.1586, 17.3712) knots 0 0 0 1 2 2 2
  spline S170 degree 2 poles (10.1586, 17.3712) (10.1883, 17.4568) (10.1377, 17.6192) (10.0451, 17.7118) knots 0 0 0 1 2 2 2
  spline S171 degree 2 poles (10.0451, 17.7118) (9.9578, 17.7991) (9.6539, 17.883) (9.4775, 17.8882) knots 0 0 0 1 2 2 2
  line L211 (9.4775, 17.8882) -> (8.2689, 16.6796)
  line L212 (8.2689, 16.6796) -> (7.9964, 16.952)
  line L213 (7.9964, 16.952) -> (9.6137, 18.5694)
  line L214 (9.6137, 18.5694) -> (9.8862, 18.2969)
  line L215 (9.8862, 18.2969) -> (9.708, 18.1187)
  spline S172 degree 2 poles (9.708, 18.1187) (9.9211, 18.1187) (10.2477, 18.0262) (10.3735, 17.9004) knots 0 0 0 1 2 2 2
  spline S173 degree 2 poles (10.3735, 17.9004) (10.5167, 17.7572) (10.6075, 17.4044) (10.5167, 17.1983) knots 0 0 0 1 2 2 2
  spline S174 degree 2 poles (10.5167, 17.1983) (10.7787, 17.2123) (11.1542, 17.1197) (11.2904, 16.9835) knots 0 0 0 1 2 2 2
  spline S175 degree 2 poles (11.2904, 16.9835) (11.3952, 16.8787) (11.5017, 16.6429) (11.4913, 16.5067) knots 0 0 0 1 2 2 2
  spline S176 degree 2 poles (11.4913, 16.5067) (11.4825, 16.3687) (11.3341, 16.077) (11.1682, 15.9111) knots 0 0 0 1 2 2 2
  line L216 (11.1682, 15.9111) -> (10.1027, 14.8457)
  line L217 (10.1027, 14.8457) -> (9.8303, 15.1181)
  spline S177 degree 2 poles (11.5576, 13.7331) (11.5, 13.7419) (11.3009, 13.7663) (11.2223, 13.7925) knots 0 0 0 1 2 2 2
  spline S178 degree 2 poles (11.2223, 13.7925) (11.1123, 13.8257) (10.9376, 13.92) (10.8153, 14.0423) knots 0 0 0 1 2 2 2
  spline S179 degree 2 poles (10.8153, 14.0423) (10.7158, 14.1418) (10.611, 14.3968) (10.611, 14.533) knots 0 0 0 1 2 2 2
  spline S180 degree 2 poles (10.611, 14.533) (10.6127, 14.664) (10.7298, 14.9382) (10.8381, 15.0465) knots 0 0 0 1 2 2 2
  spline S181 degree 2 poles (10.8381, 15.0465) (11.0057, 15.2142) (11.3847, 15.3103) (11.6065, 15.2247) knots 0 0 0 1 2 2 2
  spline S182 degree 2 poles (11.6065, 15.2247) (11.8056, 15.1513) (12.2231, 14.8282) (12.4501, 14.6256) knots 0 0 0 1 2 2 2
  line L218 (12.4501, 14.6256) -> (12.5025, 14.678)
  spline S183 degree 2 poles (12.5025, 14.678) (12.5968, 14.7723) (12.6562, 14.947) (12.637, 15.0326) knots 0 0 0 1 2 2 2
  spline S184 degree 2 poles (12.637, 15.0326) (12.6178, 15.1181) (12.4886, 15.2893) (12.4082, 15.3696) knots 0 0 0 1 2 2 2
  spline S185 degree 2 poles (12.4082, 15.3696) (12.3139, 15.464) (12.003, 15.6631) (11.8214, 15.7364) knots 0 0 0 1 2 2 2
  line L219 (11.8214, 15.7364) -> (11.8056, 15.7521)
  line L220 (11.8056, 15.7521) -> (12.0834, 16.0299)
  spline S186 degree 2 poles (12.0834, 16.0299) (12.1794, 15.9757) (12.513, 15.7469) (12.651, 15.6089) knots 0 0 0 1 2 2 2
  spline S187 degree 2 poles (12.651, 15.6089) (12.8187, 15.4413) (12.9951, 15.1601) (13.0178, 15.0011) knots 0 0 0 1 2 2 2
  spline S188 degree 2 poles (13.0178, 15.0011) (13.0405, 14.8457) (12.9165, 14.547) (12.7645, 14.3951) knots 0 0 0 1 2 2 2
  line L221 (12.7645, 14.3951) -> (11.6589, 13.2895)
  line L222 (11.6589, 13.2895) -> (11.3865, 13.562)
  line L223 (11.3865, 13.562) -> (11.5576, 13.7331)
  line L224 (11.7847, 13.9602) -> (12.2336, 14.409)
  spline S189 degree 2 poles (12.2336, 14.409) (12.127, 14.4981) (11.8022, 14.7636) (11.6816, 14.8282) knots 0 0 0 1 2 2 2
  spline S190 degree 2 poles (11.6816, 14.8282) (11.5402, 14.9033) (11.2607, 14.9068) (11.1385, 14.7845) knots 0 0 0 1 2 2 2
  spline S191 degree 2 poles (11.1385, 14.7845) (10.9987, 14.6448) (11.0145, 14.3462) (11.1647, 14.196) knots 0 0 0 1 2 2 2
  spline S192 degree 2 poles (11.1647, 14.196) (11.2922, 14.0685) (11.6118, 13.9689) (11.7847, 13.9602) knots 0 0 0 1 2 2 2
  line L225 (13.3112, 11.6372) -> (13.0387, 11.9097)
  line L226 (13.0387, 11.9097) -> (13.9609, 12.8319)
  spline S193 degree 2 poles (13.9609, 12.8319) (14.0727, 12.9437) (14.2439, 13.1568) (14.2701, 13.2458) knots 0 0 0 1 2 2 2
  spline S194 degree 2 poles (14.2701, 13.2458) (14.298, 13.3401) (14.2386, 13.5183) (14.1373, 13.6196) knots 0 0 0 1 2 2 2
  spline S195 degree 2 poles (14.1373, 13.6196) (14.036, 13.7209) (13.7129, 13.8274) (13.5225, 13.8432) knots 0 0 0 1 2 2 2
  line L227 (13.5225, 13.8432) -> (12.3139, 12.6345)
  line L228 (12.3139, 12.6345) -> (12.0414, 12.907)
  line L229 (12.0414, 12.907) -> (13.6588, 14.5243)
  line L230 (13.6588, 14.5243) -> (13.9312, 14.2518)
  line L231 (13.9312, 14.2518) -> (13.7513, 14.072)
  spline S196 degree 2 poles (13.7513, 14.072) (13.9836, 14.0597) (14.3347, 13.9392) (14.4674, 13.8065) knots 0 0 0 1 2 2 2
  spline S197 degree 2 poles (14.4674, 13.8065) (14.7049, 13.5689) (14.6595, 12.9856) (14.3609, 12.6869) knots 0 0 0 1 2 2 2
  line L232 (14.3609, 12.6869) -> (13.3112, 11.6372)
  line L233 (14.9512, 9.9972) -> (14.6787, 10.2697)
  line L234 (14.6787, 10.2697) -> (14.8569, 10.4478)
  spline S198 degree 2 poles (14.8569, 10.4478) (14.6211, 10.4635) (14.2823, 10.5753) (14.1426, 10.7151) knots 0 0 0 1 2 2 2
  spline S199 degree 2 poles (14.1426, 10.7151) (14.0378, 10.8198) (13.9207, 11.0766) (13.9277, 11.2198) knots 0 0 0 1 2 2 2
  spline S200 degree 2 poles (13.9277, 11.2198) (13.933, 11.3648) (14.0849, 11.6704) (14.2491, 11.8346) knots 0 0 0 1 2 2 2
  line L235 (14.2491, 11.8346) -> (15.2988, 12.8843)
  line L236 (15.2988, 12.8843) -> (15.5712, 12.6118)
  line L237 (15.5712, 12.6118) -> (14.6491, 11.6896)
  spline S201 degree 2 poles (14.6491, 11.6896) (14.5198, 11.5604) (14.3696, 11.3718) (14.3399, 11.2757) knots 0 0 0 1 2 2 2
  spline S202 degree 2 poles (14.3399, 11.2757) (14.3102, 11.1796) (14.3661, 11.0085) (14.4727, 10.9019) knots 0 0 0 1 2 2 2
  spline S203 degree 2 poles (14.4727, 10.9019) (14.5722, 10.8024) (14.911, 10.6906) (15.0874, 10.6784) knots 0 0 0 1 2 2 2
  line L238 (15.0874, 10.6784) -> (16.2961, 11.887)
  line L239 (16.2961, 11.887) -> (16.5685, 11.6145)
  line L240 (16.5685, 11.6145) -> (14.9512, 9.9972)
  spline S204 degree 2 poles (16.0114, 8.8637) (15.6236, 9.2514) (15.6324, 10.1125) (16.0341, 10.5142) knots 0 0 0 1 2 2 2
  spline S205 degree 2 poles (16.0341, 10.5142) (16.4288, 10.9089) (17.3108, 10.9631) (17.6444, 10.6295) knots 0 0 0 1 2 2 2
  spline S206 degree 2 poles (17.6444, 10.6295) (17.7946, 10.4793) (17.9396, 10.1596) (17.9326, 9.9815) knots 0 0 0 1 2 2 2
  spline S207 degree 2 poles (17.9326, 9.9815) (17.9274, 9.8016) (17.7527, 9.4418) (17.5588, 9.2479) knots 0 0 0 1 2 2 2
  line L241 (17.5588, 9.2479) -> (17.4104, 9.0995)
  line L242 (17.4104, 9.0995) -> (16.2908, 10.219)
  spline S208 degree 2 poles (16.2908, 10.219) (16.0096, 9.9378) (15.9939, 9.3562) (16.2454, 9.1047) knots 0 0 0 1 2 2 2
  spline S209 degree 2 poles (16.2454, 9.1047) (16.3345, 9.0156) (16.5476, 8.8829) (16.6489, 8.8445) knots 0 0 0 1 2 2 2
  spline S210 degree 2 poles (16.6489, 8.8445) (16.7572, 8.8061) (16.9196, 8.7659) (16.9807, 8.7606) knots 0 0 0 1 2 2 2
  line L243 (16.9807, 8.7606) -> (16.9964, 8.7449)
  line L244 (16.9964, 8.7449) -> (16.6995, 8.448)
  spline S211 degree 2 poles (16.6995, 8.448) (16.6332, 8.476) (16.434, 8.5633) (16.3624, 8.6035) knots 0 0 0 1 2 2 2
  spline S212 degree 2 poles (16.3624, 8.6035) (16.2611, 8.6593) (16.1092, 8.7659) (16.0114, 8.8637) knots 0 0 0 1 2 2 2
  spline S213 degree 2 poles (17.3527, 9.5728) (17.4593, 9.6863) (17.5746, 9.8924) (17.585, 9.9902) knots 0 0 0 1 2 2 2
  spline S214 degree 2 poles (17.585, 9.9902) (17.599, 10.0985) (17.5152, 10.3116) (17.4051, 10.4216) knots 0 0 0 1 2 2 2
  spline S215 degree 2 poles (17.4051, 10.4216) (17.2969, 10.5299) (17.0803, 10.6172) (16.9545, 10.6172) knots 0 0 0 1 2 2 2
  spline S216 degree 2 poles (16.9545, 10.6172) (16.8288, 10.6138) (16.6105, 10.5212) (16.4987, 10.4269) knots 0 0 0 1 2 2 2
  line L245 (16.4987, 10.4269) -> (17.3527, 9.5728)
  line L246 (17.1833, 7.7651) -> (16.9109, 8.0376)
  line L247 (16.9109, 8.0376) -> (19.1622, 10.2889)
  line L248 (19.1622, 10.2889) -> (19.4346, 10.0164)
  line L249 (19.4346, 10.0164) -> (17.1833, 7.7651)
  spline S217 degree 2 poles (18.2487, 6.6263) (17.861, 7.0141) (17.8697, 7.8751) (18.2714, 8.2768) knots 0 0 0 1 2 2 2
  spline S218 degree 2 poles (18.2714, 8.2768) (18.6662, 8.6716) (19.5482, 8.7257) (19.8818, 8.3921) knots 0 0 0 1 2 2 2
  spline S219 degree 2 poles (19.8818, 8.3921) (20.032, 8.2419) (20.1769, 7.9223) (20.17, 7.7441) knots 0 0 0 1 2 2 2
  spline S220 degree 2 poles (20.17, 7.7441) (20.1647, 7.5642) (19.9901, 7.2045) (19.7962, 7.0106) knots 0 0 0 1 2 2 2
  line L250 (19.7962, 7.0106) -> (19.6477, 6.8621)
  line L251 (19.6477, 6.8621) -> (18.5282, 7.9817)
  spline S221 degree 2 poles (18.5282, 7.9817) (18.247, 7.7005) (18.2313, 7.1189) (18.4828, 6.8674) knots 0 0 0 1 2 2 2
  spline S222 degree 2 poles (18.4828, 6.8674) (18.5718, 6.7783) (18.7849, 6.6456) (18.8862, 6.6071) knots 0 0 0 1 2 2 2
  spline S223 degree 2 poles (18.8862, 6.6071) (18.9945, 6.5687) (19.1569, 6.5285) (19.2181, 6.5233) knots 0 0 0 1 2 2 2
  line L252 (19.2181, 6.5233) -> (19.2338, 6.5076)
  line L253 (19.2338, 6.5076) -> (18.9369, 6.2107)
  spline S224 degree 2 poles (18.9369, 6.2107) (18.8705, 6.2386) (18.6714, 6.3259) (18.5998, 6.3661) knots 0 0 0 1 2 2 2
  spline S225 degree 2 poles (18.5998, 6.3661) (18.4985, 6.422) (18.3465, 6.5285) (18.2487, 6.6263) knots 0 0 0 1 2 2 2
  spline S226 degree 2 poles (19.5901, 7.3354) (19.6966, 7.449) (19.8119, 7.6551) (19.8224, 7.7529) knots 0 0 0 1 2 2 2
  spline S227 degree 2 poles (19.8224, 7.7529) (19.8364, 7.8612) (19.7525, 8.0742) (19.6425, 8.1843) knots 0 0 0 1 2 2 2
  spline S228 degree 2 poles (19.6425, 8.1843) (19.5342, 8.2926) (19.3176, 8.3799) (19.1919, 8.3799) knots 0 0 0 1 2 2 2
  spline S229 degree 2 poles (19.1919, 8.3799) (19.0661, 8.3764) (18.8478, 8.2838) (18.736, 8.1895) knots 0 0 0 1 2 2 2
  line L254 (18.736, 8.1895) -> (19.5901, 7.3354)
  spline S230 degree 2 poles (16.9237, -13.3824) (17.1578, -13.1484) (17.5839, -12.9179) (17.7988, -12.8428) knots 0 0 0 1 2 2 2
  line L255 (17.7988, -12.8428) -> (18.1586, -13.2025)
  line L256 (18.1586, -13.2025) -> (18.1376, -13.2235)
  spline S231 degree 2 poles (18.1376, -13.2235) (17.8634, -13.2322) (17.3586, -13.4436) (17.1927, -13.6095) knots 0 0 0 1 2 2 2
  spline S232 degree 2 poles (17.1927, -13.6095) (16.9552, -13.847) (16.9098, -14.2872) (17.0722, -14.4496) knots 0 0 0 1 2 2 2
  spline S233 degree 2 poles (17.0722, -14.4496) (17.2014, -14.5788) (17.4896, -14.612) (17.6678, -14.5142) knots 0 0 0 1 2 2 2
  spline S234 degree 2 poles (17.6678, -14.5142) (17.7953, -14.4426) (17.9996, -14.3151) (18.1551, -14.2225) knots 0 0 0 1 2 2 2
  spline S235 degree 2 poles (18.1551, -14.2225) (18.2965, -14.1405) (18.562, -14.0531) (18.7017, -14.0566) knots 0 0 0 1 2 2 2
  spline S236 degree 2 poles (18.7017, -14.0566) (18.8397, -14.0619) (19.1052, -14.1806) (19.231, -14.3064) knots 0 0 0 1 2 2 2
  spline S237 degree 2 poles (19.231, -14.3064) (19.4929, -14.5684) (19.4388, -15.3316) (19.1227, -15.6477) knots 0 0 0 1 2 2 2
  spline S238 degree 2 poles (19.1227, -15.6477) (18.941, -15.8294) (18.548, -16.0791) (18.342, -16.149) knots 0 0 0 1 2 2 2
  line L257 (18.342, -16.149) -> (17.9996, -15.8067)
  line L258 (17.9996, -15.8067) -> (18.0206, -15.7857)
  spline S239 degree 2 poles (18.0206, -15.7857) (18.2179, -15.777) (18.679, -15.5953) (18.8554, -15.4189) knots 0 0 0 1 2 2 2
  spline S240 degree 2 poles (18.8554, -15.4189) (19.0546, -15.2198) (19.1139, -14.7867) (18.962, -14.6347) knots 0 0 0 1 2 2 2
  spline S241 degree 2 poles (18.962, -14.6347) (18.8258, -14.4985) (18.5184, -14.481) (18.3454, -14.5806) knots 0 0 0 1 2 2 2
  spline S242 degree 2 poles (18.3454, -14.5806) (18.2302, -14.647) (17.9036, -14.8478) (17.79, -14.9089) knots 0 0 0 1 2 2 2
  spline S243 degree 2 poles (17.79, -14.9089) (17.5001, -15.0626) (17.0198, -14.9945) (16.8189, -14.7937) knots 0 0 0 1 2 2 2
  spline S244 degree 2 poles (16.8189, -14.7937) (16.6914, -14.6662) (16.55, -14.3186) (16.557, -14.1405) knots 0 0 0 1 2 2 2
  spline S245 degree 2 poles (16.557, -14.1405) (16.5657, -13.9431) (16.7264, -13.5798) (16.9237, -13.3824) knots 0 0 0 1 2 2 2
  spline S246 degree 2 poles (15.413, -16.5874) (15.0043, -16.1787) (14.9519, -15.3403) (15.2802, -15.012) knots 0 0 0 1 2 2 2
  spline S247 degree 2 poles (15.2802, -15.012) (15.6173, -14.6749) (16.4626, -14.7483) (16.8574, -15.143) knots 0 0 0 1 2 2 2
  spline S248 degree 2 poles (16.8574, -15.143) (17.2626, -15.5482) (17.3132, -16.3953) (16.9884, -16.7201) knots 0 0 0 1 2 2 2
  spline S249 degree 2 poles (16.9884, -16.7201) (16.66, -17.0485) (15.8199, -16.9943) (15.413, -16.5874) knots 0 0 0 1 2 2 2
  spline S250 degree 2 poles (15.6942, -16.3062) (16.0085, -16.6206) (16.543, -16.6974) (16.7543, -16.4861) knots 0 0 0 1 2 2 2
  spline S251 degree 2 poles (16.7543, -16.4861) (16.9657, -16.2748) (16.8906, -15.7386) (16.5762, -15.4242) knots 0 0 0 1 2 2 2
  spline S252 degree 2 poles (16.5762, -15.4242) (16.2705, -15.1185) (15.7256, -15.0347) (15.5143, -15.246) knots 0 0 0 1 2 2 2
  spline S253 degree 2 poles (15.5143, -15.246) (15.3047, -15.4556) (15.3833, -15.9953) (15.6942, -16.3062) knots 0 0 0 1 2 2 2
  spline S254 degree 2 poles (13.6454, -16.6642) (13.8131, -16.4966) (14.1939, -16.3219) (14.3982, -16.3272) knots 0 0 0 1 2 2 2
  spline S255 degree 2 poles (14.3982, -16.3272) (14.6008, -16.3306) (15.0287, -16.5385) (15.2418, -16.7516) knots 0 0 0 1 2 2 2
  spline S256 degree 2 poles (15.2418, -16.7516) (15.4549, -16.9647) (15.6522, -17.3891) (15.661, -17.5899) knots 0 0 0 1 2 2 2
  spline S257 degree 2 poles (15.661, -17.5899) (15.6715, -17.7925) (15.5003, -18.1907) (15.3361, -18.3549) knots 0 0 0 1 2 2 2
  spline S258 degree 2 poles (15.3361, -18.3549) (15.2034, -18.4877) (14.8803, -18.6606) (14.7353, -18.7077) knots 0 0 0 1 2 2 2
  line L259 (14.7353, -18.7077) -> (14.4296, -18.4021)
  line L260 (14.4296, -18.4021) -> (14.4454, -18.3864)
  spline S259 degree 2 poles (14.4454, -18.3864) (14.4995, -18.3811) (14.6532, -18.3532) (14.751, -18.3217) knots 0 0 0 1 2 2 2
  spline S260 degree 2 poles (14.751, -18.3217) (14.8366, -18.292) (15.034, -18.182) (15.1038, -18.1121) knots 0 0 0 1 2 2 2
  spline S261 degree 2 poles (15.1038, -18.1121) (15.3152, -17.9008) (15.2523, -17.3244) (14.9606, -17.0328) knots 0 0 0 1 2 2 2
  spline S262 degree 2 poles (14.9606, -17.0328) (14.6759, -16.7481) (14.1083, -16.6765) (13.8882, -16.8965) knots 0 0 0 1 2 2 2
  spline S263 degree 2 poles (13.8882, -16.8965) (13.7555, -17.0293) (13.6245, -17.3803) (13.6175, -17.5585) knots 0 0 0 1 2 2 2